Autodesk Fusion 360 part; units mm, degrees
(part 3 of 6)
  line L2235 (12.9289, -30) -> (10, -32.9289)
  line L2236 (13.3431, -31) -> (11, -33.3431)
  line L2237 (16.6569, -31) -> (13.3431, -31)
  line L2238 (19, -33.3431) -> (16.6569, -31)
  line L2239 (19, -36.6569) -> (19, -33.3431)
  line L2240 (16.6569, -39) -> (19, -36.6569)
  line L2241 (13.3431, -39) -> (16.6569, -39)
  line L2242 (11, -36.6569) -> (13.3431, -39)
  line L2243 (11, -33.3431) -> (11, -36.6569)
  line L2244 (10, -37.0711) -> (12.9289, -40)
  line L2245 (12.9289, -40) -> (17.0711, -40)
  line L2246 (17.0711, -40) -> (20, -37.0711)
  line L2247 (20, -37.0711) -> (20, -32.9289)
  line L2248 (20, -32.9289) -> (17.0711, -30)
  line L2249 (20, -32.9289) -> (20, -37.0711)
  line L2250 (22.9289, -30) -> (20, -32.9289)
  line L2251 (23.3431, -31) -> (21, -33.3431)
  line L2252 (26.6569, -31) -> (23.3431, -31)
  line L2253 (29, -33.3431) -> (26.6569, -31)
  line L2254 (29, -36.6569) -> (29, -33.3431)
  line L2255 (26.6569, -39) -> (29, -36.6569)
  line L2256 (23.3431, -39) -> (26.6569, -39)
  line L2257 (21, -36.6569) -> (23.3431, -39)
  line L2258 (21, -33.3431) -> (21, -36.6569)
  line L2259 (20, -37.0711) -> (22.9289, -40)
  line L2260 (22.9289, -40) -> (27.0711, -40)
  line L2261 (27.0711, -40) -> (30, -37.0711)
  line L2262 (30, -37.0711) -> (30, -32.9289)
  line L2263 (30, -32.9289) -> (27.0711, -30)
  line L2264 (30, -32.9289) -> (30, -37.0711)
  line L2265 (32.9289, -30) -> (30, -32.9289)
  line L2266 (33.3431, -31) -> (31, -33.3431)
  line L2267 (36.6569, -31) -> (33.3431, -31)
  line L2268 (39, -33.3431) -> (36.6569, -31)
  line L2269 (39, -36.6569) -> (39, -33.3431)
  line L2270 (36.6569, -39) -> (39, -36.6569)
  line L2271 (33.3431, -39) -> (36.6569, -39)
  line L2272 (31, -36.6569) -> (33.3431, -39)
  line L2273 (31, -33.3431) -> (31, -36.6569)
  line L2274 (30, -37.0711) -> (32.9289, -40)
  line L2275 (32.9289, -40) -> (37.0711, -40)
  line L2276 (37.0711, -40) -> (40, -37.0711)
  line L2277 (40, -37.0711) -> (40, -32.9289)
  line L2278 (40, -32.9289) -> (37.0711, -30)
  line L2279 (40, -32.9289) -> (40, -37.0711)
  line L2280 (42.9289, -30) -> (40, -32.9289)
  line L2281 (43.3431, -31) -> (41, -33.3431)
  line L2282 (46.6569, -31) -> (43.3431, -31)
  line L2283 (49, -33.3431) -> (46.6569, -31)
  line L2284 (49, -36.6569) -> (49, -33.3431)
  line L2285 (46.6569, -39) -> (49, -36.6569)
  line L2286 (43.3431, -39) -> (46.6569, -39)
  line L2287 (41, -36.6569) -> (43.3431, -39)
  line L2288 (41, -33.3431) -> (41, -36.6569)
  line L2289 (40, -37.0711) -> (42.9289, -40)
  line L2290 (42.9289, -40) -> (47.0711, -40)
  line L2291 (47.0711, -40) -> (50, -37.0711)
  line L2292 (50, -37.0711) -> (50, -32.9289)
  line L2293 (50, -32.9289) -> (47.0711, -30)
  line L2294 (50, -32.9289) -> (50, -37.0711)
  line L2295 (52.9289, -30) -> (50, -32.9289)
  line L2296 (53.3431, -31) -> (51, -33.3431)
  line L2297 (56.6569, -31) -> (53.3431, -31)
  line L2298 (59, -33.3431) -> (56.6569, -31)
  line L2299 (59, -36.6569) -> (59, -33.3431)
  line L2300 (56.6569, -39) -> (59, -36.6569)
  line L2301 (53.3431, -39) -> (56.6569, -39)
  line L2302 (51, -36.6569) -> (53.3431, -39)
  line L2303 (51, -33.3431) -> (51, -36.6569)
  line L2304 (50, -37.0711) -> (52.9289, -40)
  line L2305 (52.9289, -40) -> (57.0711, -40)
  line L2306 (57.0711, -40) -> (60, -37.0711)
  line L2307 (60, -37.0711) -> (60, -32.9289)
  line L2308 (60, -32.9289) -> (57.0711, -30)
  line L2309 (60, -32.9289) -> (60, -37.0711)
  line L2310 (62.9289, -30) -> (60, -32.9289)
  line L2311 (63.3431, -31) -> (61, -33.3431)
  line L2312 (66.6569, -31) -> (63.3431, -31)
  line L2313 (69, -33.3431) -> (66.6569, -31)
  line L2314 (69, -36.6569) -> (69, -33.3431)
  line L2315 (66.6569, -39) -> (69, -36.6569)
  line L2316 (63.3431, -39) -> (66.6569, -39)
  line L2317 (61, -36.6569) -> (63.3431, -39)
  line L2318 (61, -33.3431) -> (61, -36.6569)
  line L2319 (60, -37.0711) -> (62.9289, -40)
  line L2320 (62.9289, -40) -> (67.0711, -40)
  line L2321 (67.0711, -40) -> (70, -37.0711)
  line L2322 (70, -37.0711) -> (70, -32.9289)
  line L2323 (70, -32.9289) -> (67.0711, -30)
  line L2324 (-70, -42.9289) -> (-70, -47.0711)
  line L2325 (-67.0711, -40) -> (-70, -42.9289)
  line L2326 (-66.6569, -41) -> (-69, -43.3431)
  line L2327 (-63.3431, -41) -> (-66.6569, -41)
  line L2328 (-61, -43.3431) -> (-63.3431, -41)
  line L2329 (-61, -46.6569) -> (-61, -43.3431)
  line L2330 (-63.3431, -49) -> (-61, -46.6569)
  line L2331 (-66.6569, -49) -> (-63.3431, -49)
  line L2332 (-69, -46.6569) -> (-66.6569, -49)
  line L2333 (-69, -43.3431) -> (-69, -46.6569)
  line L2334 (-70, -47.0711) -> (-67.0711, -50)
  line L2335 (-67.0711, -50) -> (-62.9289, -50)
  line L2336 (-62.9289, -50) -> (-60, -47.0711)
  line L2337 (-60, -47.0711) -> (-60, -42.9289)
  line L2338 (-60, -42.9289) -> (-62.9289, -40)
  line L2339 (-60, -42.9289) -> (-60, -47.0711)
  line L2340 (-57.0711, -40) -> (-60, -42.9289)
  line L2341 (-56.6569, -41) -> (-59, -43.3431)
  line L2342 (-53.3431, -41) -> (-56.6569, -41)
  line L2343 (-51, -43.3431) -> (-53.3431, -41)
  line L2344 (-51, -46.6569) -> (-51, -43.3431)
  line L2345 (-53.3431, -49) -> (-51, -46.6569)
  line L2346 (-56.6569, -49) -> (-53.3431, -49)
  line L2347 (-59, -46.6569) -> (-56.6569, -49)
  line L2348 (-59, -43.3431) -> (-59, -46.6569)
  line L2349 (-60, -47.0711) -> (-57.0711, -50)
  line L2350 (-57.0711, -50) -> (-52.9289, -50)
  line L2351 (-52.9289, -50) -> (-50, -47.0711)
  line L2352 (-50, -47.0711) -> (-50, -42.9289)
  line L2353 (-50, -42.9289) -> (-52.9289, -40)
  line L2354 (-50, -42.9289) -> (-50, -47.0711)
  line L2355 (-47.0711, -40) -> (-50, -42.9289)
  line L2356 (-46.6569, -41) -> (-49, -43.3431)
  line L2357 (-43.3431, -41) -> (-46.6569, -41)
  line L2358 (-41, -43.3431) -> (-43.3431, -41)
  line L2359 (-41, -46.6569) -> (-41, -43.3431)
  line L2360 (-43.3431, -49) -> (-41, -46.6569)
  line L2361 (-46.6569, -49) -> (-43.3431, -49)
  line L2362 (-49, -46.6569) -> (-46.6569, -49)
  line L2363 (-49, -43.3431) -> (-49, -46.6569)
  line L2364 (-50, -47.0711) -> (-47.0711, -50)
  line L2365 (-47.0711, -50) -> (-42.9289, -50)
  line L2366 (-42.9289, -50) -> (-40, -47.0711)
  line L2367 (-40, -47.0711) -> (-40, -42.9289)
  line L2368 (-40, -42.9289) -> (-42.9289, -40)
  line L2369 (-40, -42.9289) -> (-40, -47.0711)
  line L2370 (-37.0711, -40) -> (-40, -42.9289)
  line L2371 (-36.6569, -41) -> (-39, -43.3431)
  line L2372 (-33.3431, -41) -> (-36.6569, -41)
  line L2373 (-31, -43.3431) -> (-33.3431, -41)
  line L2374 (-31, -46.6569) -> (-31, -43.3431)
  line L2375 (-33.3431, -49) -> (-31, -46.6569)
  line L2376 (-36.6569, -49) -> (-33.3431, -49)
  line L2377 (-39, -46.6569) -> (-36.6569, -49)
  line L2378 (-39, -43.3431) -> (-39, -46.6569)
  line L2379 (-40, -47.0711) -> (-37.0711, -50)
  line L2380 (-37.0711, -50) -> (-32.9289, -50)
  line L2381 (-32.9289, -50) -> (-30, -47.0711)
  line L2382 (-30, -47.0711) -> (-30, -42.9289)
  line L2383 (-30, -42.9289) -> (-32.9289, -40)
  line L2384 (-30, -42.9289) -> (-30, -47.0711)
  line L2385 (-27.0711, -40) -> (-30, -42.9289)
  line L2386 (-26.6569, -41) -> (-29, -43.3431)
  line L2387 (-23.3431, -41) -> (-26.6569, -41)
  line L2388 (-21, -43.3431) -> (-23.3431, -41)
  line L2389 (-21, -46.6569) -> (-21, -43.3431)
  line L2390 (-23.3431, -49) -> (-21, -46.6569)
  line L2391 (-26.6569, -49) -> (-23.3431, -49)
  line L2392 (-29, -46.6569) -> (-26.6569, -49)
  line L2393 (-29, -43.3431) -> (-29, -46.6569)
  line L2394 (-30, -47.0711) -> (-27.0711, -50)
  line L2395 (-27.0711, -50) -> (-22.9289, -50)
  line L2396 (-22.9289, -50) -> (-20, -47.0711)
  line L2397 (-20, -47.0711) -> (-20, -42.9289)
  line L2398 (-20, -42.9289) -> (-22.9289, -40)
  line L2399 (-20, -42.9289) -> (-20, -47.0711)
  line L2400 (-17.0711, -40) -> (-20, -42.9289)
  line L2401 (-16.6569, -41) -> (-19, -43.3431)
  line L2402 (-13.3431, -41) -> (-16.6569, -41)
  line L2403 (-11, -43.3431) -> (-13.3431, -41)
  line L2404 (-11, -46.6569) -> (-11, -43.3431)
  line L2405 (-13.3431, -49) -> (-11, -46.6569)
  line L2406 (-16.6569, -49) -> (-13.3431, -49)
  line L2407 (-19, -46.6569) -> (-16.6569, -49)
  line L2408 (-19, -43.3431) -> (-19, -46.6569)
  line L2409 (-20, -47.0711) -> (-17.0711, -50)
  line L2410 (-17.0711, -50) -> (-12.9289, -50)
  line L2411 (-12.9289, -50) -> (-10, -47.0711)
  line L2412 (-10, -47.0711) -> (-10, -42.9289)
  line L2413 (-10, -42.9289) -> (-12.9289, -40)
  line L2414 (-10, -42.9289) -> (-10, -47.0711)
  line L2415 (-7.0711, -40) -> (-10, -42.9289)
  line L2416 (-6.6569, -41) -> (-9, -43.3431)
  line L2417 (-3.3431, -41) -> (-6.6569, -41)
  line L2418 (-1, -43.3431) -> (-3.3431, -41)
  line L2419 (-1, -46.6569) -> (-1, -43.3431)
  line L2420 (-3.3431, -49) -> (-1, -46.6569)
  line L2421 (-6.6569, -49) -> (-3.3431, -49)
  line L2422 (-9, -46.6569) -> (-6.6569, -49)
  line L2423 (-9, -43.3431) -> (-9, -46.6569)
  line L2424 (-10, -47.0711) -> (-7.0711, -50)
  line L2425 (-7.0711, -50) -> (-2.9289, -50)
  line L2426 (-2.9289, -50) -> (0, -47.0711)
  line L2427 (0, -47.0711) -> (0, -42.9289)
  line L2428 (0, -42.9289) -> (-2.9289, -40)
  line L2429 (0, -42.9289) -> (0, -47.0711)
  line L2430 (2.9289, -40) -> (0, -42.9289)
  line L2431 (3.3431, -41) -> (1, -43.3431)
  line L2432 (6.6569, -41) -> (3.3431, -41)
  line L2433 (9, -43.3431) -> (6.6569, -41)
  line L2434 (9, -46.6569) -> (9, -43.3431)
  line L2435 (6.6569, -49) -> (9, -46.6569)
  line L2436 (3.3431, -49) -> (6.6569, -49)
  line L2437 (1, -46.6569) -> (3.3431, -49)
  line L2438 (1, -43.3431) -> (1, -46.6569)
  line L2439 (0, -47.0711) -> (2.9289, -50)
  line L2440 (2.9289, -50) -> (7.0711, -50)
  line L2441 (7.0711, -50) -> (10, -47.0711)
  line L2442 (10, -47.0711) -> (10, -42.9289)
  line L2443 (10, -42.9289) -> (7.0711, -40)
  line L2444 (10, -42.9289) -> (10, -47.0711)
  line L2445 (12.9289, -40) -> (10, -42.9289)
  line L2446 (13.3431, -41) -> (11, -43.3431)
  line L2447 (16.6569, -41) -> (13.3431, -41)
  line L2448 (19, -43.3431) -> (16.6569, -41)
  line L2449 (19, -46.6569) -> (19, -43.3431)
  line L2450 (16.6569, -49) -> (19, -46.6569)
  line L2451 (13.3431, -49) -> (16.6569, -49)
  line L2452 (11, -46.6569) -> (13.3431, -49)
  line L2453 (11, -43.3431) -> (11, -46.6569)
  line L2454 (10, -47.0711) -> (12.9289, -50)
  line L2455 (12.9289, -50) -> (17.0711, -50)
  line L2456 (17.0711, -50) -> (20, -47.0711)
  line L2457 (20, -47.0711) -> (20, -42.9289)
  line L2458 (20, -42.9289) -> (17.0711, -40)
  line L2459 (20, -42.9289) -> (20, -47.0711)
  line L2460 (22.9289, -40) -> (20, -42.9289)
  line L2461 (23.3431, -41) -> (21, -43.3431)
  line L2462 (26.6569, -41) -> (23.3431, -41)
  line L2463 (29, -43.3431) -> (26.6569, -41)
  line L2464 (29, -46.6569) -> (29, -43.3431)
  line L2465 (26.6569, -49) -> (29, -46.6569)
  line L2466 (23.3431, -49) -> (26.6569, -49)
  line L2467 (21, -46.6569) -> (23.3431, -49)
  line L2468 (21, -43.3431) -> (21, -46.6569)
  line L2469 (20, -47.0711) -> (22.9289, -50)
  line L2470 (22.9289, -50) -> (27.0711, -50)
  line L2471 (27.0711, -50) -> (30, -47.0711)
  line L2472 (30, -47.0711) -> (30, -42.9289)
  line L2473 (30, -42.9289) -> (27.0711, -40)
  line L2474 (30, -42.9289) -> (30, -47.0711)
  line L2475 (32.9289, -40) -> (30, -42.9289)
  line L2476 (33.3431, -41) -> (31, -43.3431)
  line L2477 (36.6569, -41) -> (33.3431, -41)
  line L2478 (39, -43.3431) -> (36.6569, -41)
  line L2479 (39, -46.6569) -> (39, -43.3431)
  line L2480 (36.6569, -49) -> (39, -46.6569)
  line L2481 (33.3431, -49) -> (36.6569, -49)
  line L2482 (31, -46.6569) -> (33.3431, -49)
  line L2483 (31, -43.3431) -> (31, -46.6569)
  line L2484 (30, -47.0711) -> (32.9289, -50)
  line L2485 (32.9289, -50) -> (37.0711, -50)
  line L2486 (37.0711, -50) -> (40, -47.0711)
  line L2487 (40, -47.0711) -> (40, -42.9289)
  line L2488 (40, -42.9289) -> (37.0711, -40)
  line L2489 (40, -42.9289) -> (40, -47.0711)
  line L2490 (42.9289, -40) -> (40, -42.9289)
  line L2491 (43.3431, -41) -> (41, -43.3431)
  line L2492 (46.6569, -41) -> (43.3431, -41)
  line L2493 (49, -43.3431) -> (46.6569, -41)
  line L2494 (49, -46.6569) -> (49, -43.3431)
  line L2495 (46.6569, -49) -> (49, -46.6569)
  line L2496 (43.3431, -49) -> (46.6569, -49)
  line L2497 (41, -46.6569) -> (43.3431, -49)
  line L2498 (41, -43.3431) -> (41, -46.6569)
  line L2499 (40, -47.0711) -> (42.9289, -50)
  line L2500 (42.9289, -50) -> (47.0711, -50)
  line L2501 (47.0711, -50) -> (50, -47.0711)
  line L2502 (50, -47.0711) -> (50, -42.9289)
  line L2503 (50, -42.9289) -> (47.0711, -40)
  line L2504 (50, -42.9289) -> (50, -47.0711)
  line L2505 (52.9289, -40) -> (50, -42.9289)
  line L2506 (53.3431, -41) -> (51, -43.3431)
  line L2507 (56.6569, -41) -> (53.3431, -41)
  line L2508 (59, -43.3431) -> (56.6569, -41)
  line L2509 (59, -46.6569) -> (59, -43.3431)
  line L2510 (56.6569, -49) -> (59, -46.6569)
  line L2511 (53.3431, -49) -> (56.6569, -49)
  line L2512 (51, -46.6569) -> (53.3431, -49)
  line L2513 (51, -43.3431) -> (51, -46.6569)
  line L2514 (50, -47.0711) -> (52.9289, -50)
  line L2515 (52.9289, -50) -> (57.0711, -50)
  line L2516 (57.0711, -50) -> (60, -47.0711)
  line L2517 (60, -47.0711) -> (60, -42.9289)
  line L2518 (60, -42.9289) -> (57.0711, -40)
  line L2519 (60, -42.9289) -> (60, -47.0711)
  line L2520 (62.9289, -40) -> (60, -42.9289)
  line L2521 (63.3431, -41) -> (61, -43.3431)
  line L2522 (66.6569, -41) -> (63.3431, -41)
  line L2523 (69, -43.3431) -> (66.6569, -41)
  line L2524 (69, -46.6569) -> (69, -43.3431)
  line L2525 (66.6569, -49) -> (69, -46.6569)
  line L2526 (63.3431, -49) -> (66.6569, -49)
  line L2527 (61, -46.6569) -> (63.3431, -49)
  line L2528 (61, -43.3431) -> (61, -46.6569)
  line L2529 (60, -47.0711) -> (62.9289, -50)
  line L2530 (62.9289, -50) -> (67.0711, -50)
  line L2531 (67.0711, -50) -> (70, -47.0711)
  line L2532 (70, -47.0711) -> (70, -42.9289)
  line L2533 (70, -42.9289) -> (67.0711, -40)
  line L2534 (-70, -52.9289) -> (-70, -57.0711)
  line L2535 (-67.0711, -50) -> (-70, -52.9289)
  line L2536 (-66.6569, -51) -> (-69, -53.3431)
  line L2537 (-63.3431, -51) -> (-66.6569, -51)
  line L2538 (-61, -53.3431) -> (-63.3431, -51)
  line L2539 (-61, -56.6569) -> (-61, -53.3431)
  line L2540 (-63.3431, -59) -> (-61, -56.6569)
  line L2541 (-66.6569, -59) -> (-63.3431, -59)
  line L2542 (-69, -56.6569) -> (-66.6569, -59)
  line L2543 (-69, -53.3431) -> (-69, -56.6569)
  line L2544 (-70, -57.0711) -> (-67.0711, -60)
  line L2545 (-67.0711, -60) -> (-62.9289, -60)
  line L2546 (-62.9289, -60) -> (-60, -57.0711)
  line L2547 (-60, -57.0711) -> (-60, -52.9289)
  line L2548 (-60, -52.9289) -> (-62.9289, -50)
  line L2549 (-60, -52.9289) -> (-60, -57.0711)
  line L2550 (-57.0711, -50) -> (-60, -52.9289)
  line L2551 (-56.6569, -51) -> (-59, -53.3431)
  line L2552 (-53.3431, -51) -> (-56.6569, -51)
  line L2553 (-51, -53.3431) -> (-53.3431, -51)
  line L2554 (-51, -56.6569) -> (-51, -53.3431)
  line L2555 (-53.3431, -59) -> (-51, -56.6569)
  line L2556 (-56.6569, -59) -> (-53.3431, -59)
  line L2557 (-59, -56.6569) -> (-56.6569, -59)
  line L2558 (-59, -53.3431) -> (-59, -56.6569)
  line L2559 (-60, -57.0711) -> (-57.0711, -60)
  line L2560 (-57.0711, -60) -> (-52.9289, -60)
  line L2561 (-52.9289, -60) -> (-50, -57.0711)
  line L2562 (-50, -57.0711) -> (-50, -52.9289)
  line L2563 (-50, -52.9289) -> (-52.9289, -50)
  line L2564 (-50, -52.9289) -> (-50, -57.0711)
  line L2565 (-47.0711, -50) -> (-50, -52.9289)
  line L2566 (-46.6569, -51) -> (-49, -53.3431)
  line L2567 (-43.3431, -51) -> (-46.6569, -51)
  line L2568 (-41, -53.3431) -> (-43.3431, -51)
  line L2569 (-41, -56.6569) -> (-41, -53.3431)
  line L2570 (-43.3431, -59) -> (-41, -56.6569)
  line L2571 (-46.6569, -59) -> (-43.3431, -59)
  line L2572 (-49, -56.6569) -> (-46.6569, -59)
  line L2573 (-49, -53.3431) -> (-49, -56.6569)
  line L2574 (-50, -57.0711) -> (-47.0711, -60)
  line L2575 (-47.0711, -60) -> (-42.9289, -60)
  line L2576 (-42.9289, -60) -> (-40, -57.0711)
  line L2577 (-40, -57.0711) -> (-40, -52.9289)
  line L2578 (-40, -52.9289) -> (-42.9289, -50)
  line L2579 (-40, -52.9289) -> (-40, -57.0711)
  line L2580 (-37.0711, -50) -> (-40, -52.9289)
  line L2581 (-36.6569, -51) -> (-39, -53.3431)
  line L2582 (-33.3431, -51) -> (-36.6569, -51)
  line L2583 (-31, -53.3431) -> (-33.3431, -51)
  line L2584 (-31, -56.6569) -> (-31, -53.3431)
  line L2585 (-33.3431, -59) -> (-31, -56.6569)
  line L2586 (-36.6569, -59) -> (-33.3431, -59)
  line L2587 (-39, -56.6569) -> (-36.6569, -59)
  line L2588 (-39, -53.3431) -> (-39, -56.6569)
  line L2589 (-40, -57.0711) -> (-37.0711, -60)
  line L2590 (-37.0711, -60) -> (-32.9289, -60)
  line L2591 (-32.9289, -60) -> (-30, -57.0711)
  line L2592 (-30, -57.0711) -> (-30, -52.9289)
  line L2593 (-30, -52.9289) -> (-32.9289, -50)
  line L2594 (-30, -52.9289) -> (-30, -57.0711)
  line L2595 (-27.0711, -50) -> (-30, -52.9289)
  line L2596 (-26.6569, -51) -> (-29, -53.3431)
  line L2597 (-23.3431, -51) -> (-26.6569, -51)
  line L2598 (-21, -53.3431) -> (-23.3431, -51)
  line L2599 (-21, -56.6569) -> (-21, -53.3431)
  line L2600 (-23.3431, -59) -> (-21, -56.6569)
  line L2601 (-26.6569, -59) -> (-23.3431, -59)
  line L2602 (-29, -56.6569) -> (-26.6569, -59)
  line L2603 (-29, -53.3431) -> (-29, -56.6569)
  line L2604 (-30, -57.0711) -> (-27.0711, -60)
  line L2605 (-27.0711, -60) -> (-22.9289, -60)
  line L2606 (-22.9289, -60) -> (-20, -57.0711)
  line L2607 (-20, -57.0711) -> (-20, -52.9289)
  line L2608 (-20, -52.9289) -> (-22.9289, -50)
  line L2609 (-20, -52.9289) -> (-20, -57.0711)
  line L2610 (-17.0711, -50) -> (-20, -52.9289)
  line L2611 (-16.6569, -51) -> (-19, -53.3431)
  line L2612 (-13.3431, -51) -> (-16.6569, -51)
  line L2613 (-11, -53.3431) -> (-13.3431, -51)
  line L2614 (-11, -56.6569) -> (-11, -53.3431)
  line L2615 (-13.3431, -59) -> (-11, -56.6569)
  line L2616 (-16.6569, -59) -> (-13.3431, -59)
  line L2617 (-19, -56.6569) -> (-16.6569, -59)
  line L2618 (-19, -53.3431) -> (-19, -56.6569)
  line L2619 (-20, -57.0711) -> (-17.0711, -60)
  line L2620 (-17.0711, -60) -> (-12.9289, -60)
  line L2621 (-12.9289, -60) -> (-10, -57.0711)
  line L2622 (-10, -57.0711) -> (-10, -52.9289)
  line L2623 (-10, -52.9289) -> (-12.9289, -50)
  line L2624 (-10, -52.9289) -> (-10, -57.0711)
  line L2625 (-7.0711, -50) -> (-10, -52.9289)
  line L2626 (-6.6569, -51) -> (-9, -53.3431)
  line L2627 (-3.3431, -51) -> (-6.6569, -51)
  line L2628 (-1, -53.3431) -> (-3.3431, -51)
  line L2629 (-1, -56.6569) -> (-1, -53.3431)
  line L2630 (-3.3431, -59) -> (-1, -56.6569)
  line L2631 (-6.6569, -59) -> (-3.3431, -59)
  line L2632 (-9, -56.6569) -> (-6.6569, -59)
  line L2633 (-9, -53.3431) -> (-9, -56.6569)
  line L2634 (-10, -57.0711) -> (-7.0711, -60)
  line L2635 (-7.0711, -60) -> (-2.9289, -60)
  line L2636 (-2.9289, -60) -> (0, -57.0711)
  line L2637 (0, -57.0711) -> (0, -52.9289)
  line L2638 (0, -52.9289) -> (-2.9289, -50)
  line L2639 (0, -52.9289) -> (0, -57.0711)
  line L2640 (2.9289, -50) -> (0, -52.9289)
  line L2641 (3.3431, -51) -> (1, -53.3431)
  line L2642 (6.6569, -51) -> (3.3431, -51)
  line L2643 (9, -53.3431) -> (6.6569, -51)
  line L2644 (9, -56.6569) -> (9, -53.3431)
  line L2645 (6.6569, -59) -> (9, -56.6569)
  line L2646 (3.3431, -59) -> (6.6569, -59)
  line L2647 (1, -56.6569) -> (3.3431, -59)
  line L2648 (1, -53.3431) -> (1, -56.6569)
  line L2649 (0, -57.0711) -> (2.9289, -60)
  line L2650 (2.9289, -60) -> (7.0711, -60)
  line L2651 (7.0711, -60) -> (10, -57.0711)
  line L2652 (10, -57.0711) -> (10, -52.9289)
  line L2653 (10, -52.9289) -> (7.0711, -50)
  line L2654 (10, -52.9289) -> (10, -57.0711)
  line L2655 (12.9289, -50) -> (10, -52.9289)
  line L2656 (13.3431, -51) -> (11, -53.3431)
  line L2657 (16.6569, -51) -> (13.3431, -51)
  line L2658 (19, -53.3431) -> (16.6569, -51)
  line L2659 (19, -56.6569) -> (19, -53.3431)
  line L2660 (16.6569, -59) -> (19, -56.6569)
  line L2661 (13.3431, -59) -> (16.6569, -59)
  line L2662 (11, -56.6569) -> (13.3431, -59)
  line L2663 (11, -53.3431) -> (11, -56.6569)
  line L2664 (10, -57.0711) -> (12.9289, -60)
  line L2665 (12.9289, -60) -> (17.0711, -60)
  line L2666 (17.0711, -60) -> (20, -57.0711)
  line L2667 (20, -57.0711) -> (20, -52.9289)
  line L2668 (20, -52.9289) -> (17.0711, -50)
  line L2669 (20, -52.9289) -> (20, -57.0711)
  line L2670 (22.9289, -50) -> (20, -52.9289)
  line L2671 (23.3431, -51) -> (21, -53.3431)
  line L2672 (26.6569, -51) -> (23.3431, -51)
  line L2673 (29, -53.3431) -> (26.6569, -51)
  line L2674 (29, -56.6569) -> (29, -53.3431)
  line L2675 (26.6569, -59) -> (29, -56.6569)
  line L2676 (23.3431, -59) -> (26.6569, -59)
  line L2677 (21, -56.6569) -> (23.3431, -59)
  line L2678 (21, -53.3431) -> (21, -56.6569)
  line L2679 (20, -57.0711) -> (22.9289, -60)
  line L2680 (22.9289, -60) -> (27.0711, -60)
  line L2681 (27.0711, -60) -> (30, -57.0711)
  line L2682 (30, -57.0711) -> (30, -52.9289)
  line L2683 (30, -52.9289) -> (27.0711, -50)
  line L2684 (30, -52.9289) -> (30, -57.0711)
  line L2685 (32.9289, -50) -> (30, -52.9289)
  line L2686 (33.3431, -51) -> (31, -53.3431)
  line L2687 (36.6569, -51) -> (33.3431, -51)
  line L2688 (39, -53.3431) -> (36.6569, -51)
  line L2689 (39, -56.6569) -> (39, -53.3431)
  line L2690 (36.6569, -59) -> (39, -56.6569)
  line L2691 (33.3431, -59) -> (36.6569, -59)
  line L2692 (31, -56.6569) -> (33.3431, -59)
  line L2693 (31, -53.3431) -> (31, -56.6569)
  line L2694 (30, -57.0711) -> (32.9289, -60)
  line L2695 (32.9289, -60) -> (37.0711, -60)
  line L2696 (37.0711, -60) -> (40, -57.0711)
  line L2697 (40, -57.0711) -> (40, -52.9289)
  line L2698 (40, -52.9289) -> (37.0711, -50)
  line L2699 (40, -52.9289) -> (40, -57.0711)
  line L2700 (42.9289, -50) -> (40, -52.9289)
  line L2701 (43.3431, -51) -> (41, -53.3431)
  line L2702 (46.6569, -51) -> (43.3431, -51)
  line L2703 (49, -53.3431) -> (46.6569, -51)
  line L2704 (49, -56.6569) -> (49, -53.3431)
  line L2705 (46.6569, -59) -> (49, -56.6569)
  line L2706 (43.3431, -59) -> (46.6569, -59)
  line L2707 (41, -56.6569) -> (43.3431, -59)
  line L2708 (41, -53.3431) -> (41, -56.6569)
  line L2709 (40, -57.0711) -> (42.9289, -60)
  line L2710 (42.9289, -60) -> (47.0711, -60)
  line L2711 (47.0711, -60) -> (50, -57.0711)
  line L2712 (50, -57.0711) -> (50, -52.9289)
  line L2713 (50, -52.9289) -> (47.0711, -50)
  line L2714 (50, -52.9289) -> (50, -57.0711)
  line L2715 (52.9289, -50) -> (50, -52.9289)
  line L2716 (53.3431, -51) -> (51, -53.3431)
  line L2717 (56.6569, -51) -> (53.3431, -51)
  line L2718 (59, -53.3431) -> (56.6569, -51)
  line L2719 (59, -56.6569) -> (59, -53.3431)
  line L2720 (56.6569, -59) -> (59, -56.6569)
  line L2721 (53.3431, -59) -> (56.6569, -59)
  line L2722 (51, -56.6569) -> (53.3431, -59)
  line L2723 (51, -53.3431) -> (51, -56.6569)
  line L2724 (50, -57.0711) -> (52.9289, -60)
  line L2725 (52.9289, -60) -> (57.0711, -60)
  line L2726 (57.0711, -60) -> (60, -57.0711)
  line L2727 (60, -57.0711) -> (60, -52.9289)
  line L2728 (60, -52.9289) -> (57.0711, -50)
  line L2729 (60, -52.9289) -> (60, -57.0711)
  line L2730 (62.9289, -50) -> (60, -52.9289)
  line L2731 (63.3431, -51) -> (61, -53.3431)
  line L2732 (66.6569, -51) -> (63.3431, -51)
  line L2733 (69, -53.3431) -> (66.6569, -51)
  line L2734 (69, -56.6569) -> (69, -53.3431)
  line L2735 (66.6569, -59) -> (69, -56.6569)
  line L2736 (63.3431, -59) -> (66.6569, -59)
  line L2737 (61, -56.6569) -> (63.3431, -59)
  line L2738 (61, -53.3431) -> (61, -56.6569)
  line L2739 (60, -57.0711) -> (62.9289, -60)
  line L2740 (62.9289, -60) -> (67.0711, -60)
  line L2741 (67.0711, -60) -> (70, -57.0711)
  line L2742 (70, -57.0711) -> (70, -52.9289)
  line L2743 (70, -52.9289) -> (67.0711, -50)
  line L2744 (-70, -62.9289) -> (-70, -67.0711)
  line L2745 (-67.0711, -60) -> (-70, -62.9289)
  line L2746 (-66.6569, -61) -> (-69, -63.3431)
  line L2747 (-63.3431, -61) -> (-66.6569, -61)
  line L2748 (-61, -63.3431) -> (-63.3431, -61)
  line L2749 (-61, -66.6569) -> (-61, -63.3431)
  line L2750 (-63.3431, -69) -> (-61, -66.6569)
  line L2751 (-66.6569, -69) -> (-63.3431, -69)
  line L2752 (-69, -66.6569) -> (-66.6569, -69)
  line L2753 (-69, -63.3431) -> (-69, -66.6569)
  line L2754 (-70, -67.0711) -> (-67.0711, -70)
  line L2755 (-67.0711, -70) -> (-62.9289, -70)
  line L2756 (-62.9289, -70) -> (-60, -67.0711)
  line L2757 (-60, -67.0711) -> (-60, -62.9289)
  line L2758 (-60, -62.9289) -> (-62.9289, -60)
  line L2759 (-60, -62.9289) -> (-60, -67.0711)
  line L2760 (-57.0711, -60) -> (-60, -62.9289)
  line L2761 (-56.6569, -61) -> (-59, -63.3431)
  line L2762 (-53.3431, -61) -> (-56.6569, -61)
  line L2763 (-51, -63.3431) -> (-53.3431, -61)
  line L2764 (-51, -66.6569) -> (-51, -63.3431)
  line L2765 (-53.3431, -69) -> (-51, -66.6569)
  line L2766 (-56.6569, -69) -> (-53.3431, -69)
  line L2767 (-59, -66.6569) -> (-56.6569, -69)
  line L2768 (-59, -63.3431) -> (-59, -66.6569)
  line L2769 (-60, -67.0711) -> (-57.0711, -70)
  line L2770 (-57.0711, -70) -> (-52.9289, -70)
  line L2771 (-52.9289, -70) -> (-50, -67.0711)
  line L2772 (-50, -67.0711) -> (-50, -62.9289)
  line L2773 (-50, -62.9289) -> (-52.9289, -60)
  line L2774 (-50, -62.9289) -> (-50, -67.0711)
  line L2775 (-47.0711, -60) -> (-50, -62.9289)
  line L2776 (-46.6569, -61) -> (-49, -63.3431)
  line L2777 (-43.3431, -61) -> (-46.6569, -61)
  line L2778 (-41, -63.3431) -> (-43.3431, -61)
  line L2779 (-41, -66.6569) -> (-41, -63.3431)
  line L2780 (-43.3431, -69) -> (-41, -66.6569)
  line L2781 (-46.6569, -69) -> (-43.3431, -69)
  line L2782 (-49, -66.6569) -> (-46.6569, -69)
  line L2783 (-49, -63.3431) -> (-49, -66.6569)
  line L2784 (-50, -67.0711) -> (-47.0711, -70)
  line L2785 (-47.0711, -70) -> (-42.9289, -70)
  line L2786 (-42.9289, -70) -> (-40, -67.0711)
  line L2787 (-40, -67.0711) -> (-40, -62.9289)
  line L2788 (-40, -62.9289) -> (-42.9289, -60)
  line L2789 (-40, -62.9289) -> (-40, -67.0711)
  line L2790 (-37.0711, -60) -> (-40, -62.9289)
  line L2791 (-36.6569, -61) -> (-39, -63.3431)
  line L2792 (-33.3431, -61) -> (-36.6569, -61)
  line L2793 (-31, -63.3431) -> (-33.3431, -61)
  line L2794 (-31, -66.6569) -> (-31, -63.3431)
  line L2795 (-33.3431, -69) -> (-31, -66.6569)
  line L2796 (-36.6569, -69) -> (-33.3431, -69)
  line L2797 (-39, -66.6569) -> (-36.6569, -69)
  line L2798 (-39, -63.3431) -> (-39, -66.6569)
  line L2799 (-40, -67.0711) -> (-37.0711, -70)
  line L2800 (-37.0711, -70) -> (-32.9289, -70)
  line L2801 (-32.9289, -70) -> (-30, -67.0711)
  line L2802 (-30, -67.0711) -> (-30, -62.9289)
  line L2803 (-30, -62.9289) -> (-32.9289, -60)
  line L2804 (-30, -62.9289) -> (-30, -67.0711)
  line L2805 (-27.0711, -60) -> (-30, -62.9289)
  line L2806 (-26.6569, -61) -> (-29, -63.3431)
  line L2807 (-23.3431, -61) -> (-26.6569, -61)
  line L2808 (-21, -63.3431) -> (-23.3431, -61)
  line L2809 (-21, -66.6569) -> (-21, -63.3431)
  line L2810 (-23.3431, -69) -> (-21, -66.6569)
  line L2811 (-26.6569, -69) -> (-23.3431, -69)
  line L2812 (-29, -66.6569) -> (-26.6569, -69)
  line L2813 (-29, -63.3431) -> (-29, -66.6569)
  line L2814 (-30, -67.0711) -> (-27.0711, -70)
  line L2815 (-27.0711, -70) -> (-22.9289, -70)
  line L2816 (-22.9289, -70) -> (-20, -67.0711)
  line L2817 (-20, -67.0711) -> (-20, -62.9289)
  line L2818 (-20, -62.9289) -> (-22.9289, -60)
  line L2819 (-20, -62.9289) -> (-20, -67.0711)
  line L2820 (-17.0711, -60) -> (-20, -62.9289)
  line L2821 (-16.6569, -61) -> (-19, -63.3431)
  line L2822 (-13.3431, -61) -> (-16.6569, -61)
  line L2823 (-11, -63.3431) -> (-13.3431, -61)
  line L2824 (-11, -66.6569) -> (-11, -63.3431)
  line L2825 (-13.3431, -69) -> (-11, -66.6569)
  line L2826 (-16.6569, -69) -> (-13.3431, -69)
  line L2827 (-19, -66.6569) -> (-16.6569, -69)
  line L2828 (-19, -63.3431) -> (-19, -66.6569)
  line L2829 (-20, -67.0711) -> (-17.0711, -70)
  line L2830 (-17.0711, -70) -> (-12.9289, -70)
  line L2831 (-12.9289, -70) -> (-10, -67.0711)
  line L2832 (-10, -67.0711) -> (-10, -62.9289)
  line L2833 (-10, -62.9289) -> (-12.9289, -60)
  line L2834 (-10, -62.9289) -> (-10, -67.0711)
  line L2835 (-7.0711, -60) -> (-10, -62.9289)
  line L2836 (-6.6569, -61) -> (-9, -63.3431)
  line L2837 (-3.3431, -61) -> (-6.6569, -61)
  line L2838 (-1, -63.3431) -> (-3.3431, -61)
  line L2839 (-1, -66.6569) -> (-1, -63.3431)
  line L2840 (-3.3431, -69) -> (-1, -66.6569)
  line L2841 (-6.6569, -69) -> (-3.3431, -69)
  line L2842 (-9, -66.6569) -> (-6.6569, -69)
  line L2843 (-9, -63.3431) -> (-9, -66.6569)
  line L2844 (-10, -67.0711) -> (-7.0711, -70)
  line L2845 (-7.0711, -70) -> (-2.9289, -70)
  line L2846 (-2.9289, -70) -> (0, -67.0711)
  line L2847 (0, -67.0711) -> (0, -62.9289)
  line L2848 (0, -62.9289) -> (-2.9289, -60)
  line L2849 (0, -62.9289) -> (0, -67.0711)
  line L2850 (2.9289, -60) -> (0, -62.9289)
  line L2851 (3.3431, -61) -> (1, -63.3431)
  line L2852 (6.6569, -61) -> (3.3431, -61)
  line L2853 (9, -63.3431) -> (6.6569, -61)
  line L2854 (9, -66.6569) -> (9, -63.3431)
  line L2855 (6.6569, -69) -> (9, -66.6569)
  line L2856 (3.3431, -69) -> (6.6569, -69)
  line L2857 (1, -66.6569) -> (3.3431, -69)
  line L2858 (1, -63.3431) -> (1, -66.6569)
  line L2859 (0, -67.0711) -> (2.9289, -70)
  line L2860 (2.9289, -70) -> (7.0711, -70)
  line L2861 (7.0711, -70) -> (10, -67.0711)
  line L2862 (10, -67.0711) -> (10, -62.9289)
  line L2863 (10, -62.9289) -> (7.0711, -60)
  line L2864 (10, -62.9289) -> (10, -67.0711)
  line L2865 (12.9289, -60) -> (10, -62.9289)
  line L2866 (13.3431, -61) -> (11, -63.3431)
  line L2867 (16.6569, -61) -> (13.3431, -61)
  line L2868 (19, -63.3431) -> (16.6569, -61)
  line L2869 (19, -66.6569) -> (19, -63.3431)
  line L2870 (16.6569, -69) -> (19, -66.6569)
  line L2871 (13.3431, -69) -> (16.6569, -69)
  line L2872 (11, -66.6569) -> (13.3431, -69)
  line L2873 (11, -63.3431) -> (11, -66.6569)
  line L2874 (10, -67.0711) -> (12.9289, -70)
  line L2875 (12.9289, -70) -> (17.0711, -70)
  line L2876 (17.0711, -70) -> (20, -67.0711)
  line L2877 (20, -67.0711) -> (20, -62.9289)
  line L2878 (20, -62.9289) -> (17.0711, -60)
  line L2879 (20, -62.9289) -> (20, -67.0711)
  line L2880 (22.9289, -60) -> (20, -62.9289)
  line L2881 (23.3431, -61) -> (21, -63.3431)
  line L2882 (26.6569, -61) -> (23.3431, -61)
  line L2883 (29, -63.3431) -> (26.6569, -61)
  line L2884 (29, -66.6569) -> (29, -63.3431)
  line L2885 (26.6569, -69) -> (29, -66.6569)
  line L2886 (23.3431, -69) -> (26.6569, -69)
  line L2887 (21, -66.6569) -> (23.3431, -69)
  line L2888 (21, -63.3431) -> (21, -66.6569)
  line L2889 (20, -67.0711) -> (22.9289, -70)
  line L2890 (22.9289, -70) -> (27.0711, -70)
  line L2891 (27.0711, -70) -> (30, -67.0711)
  line L2892 (30, -67.0711) -> (30, -62.9289)
  line L2893 (30, -62.9289) -> (27.0711, -60)
  line L2894 (30, -62.9289) -> (30, -67.0711)
  line L2895 (32.9289, -60) -> (30, -62.9289)
  line L2896 (33.3431, -61) -> (31, -63.3431)
  line L2897 (36.6569, -61) -> (33.3431, -61)
  line L2898 (39, -63.3431) -> (36.6569, -61)
  line L2899 (39, -66.6569) -> (39, -63.3431)
  line L2900 (36.6569, -69) -> (39, -66.6569)
  line L2901 (33.3431, -69) -> (36.6569, -69)
  line L2902 (31, -66.6569) -> (33.3431, -69)
  line L2903 (31, -63.3431) -> (31, -66.6569)
  line L2904 (30, -67.0711) -> (32.9289, -70)
  line L2905 (32.9289, -70) -> (37.0711, -70)
  line L2906 (37.0711, -70) -> (40, -67.0711)
  line L2907 (40, -67.0711) -> (40, -62.9289)
  line L2908 (40, -62.9289) -> (37.0711, -60)
  line L2909 (40, -62.9289) -> (40, -67.0711)
  line L2910 (42.9289, -60) -> (40, -62.9289)
  line L2911 (43.3431, -61) -> (41, -63.3431)
  line L2912 (46.6569, -61) -> (43.3431, -61)
  line L2913 (49, -63.3431) -> (46.6569, -61)
  line L2914 (49, -66.6569) -> (49, -63.3431)
  line L2915 (46.6569, -69) -> (49, -66.6569)
  line L2916 (43.3431, -69) -> (46.6569, -69)
  line L2917 (41, -66.6569) -> (43.3431, -69)
  line L2918 (41, -63.3431) -> (41, -66.6569)
  line L2919 (40, -67.0711) -> (42.9289, -70)
  line L2920 (42.9289, -70) -> (47.0711, -70)
  line L2921 (47.0711, -70) -> (50, -67.0711)
  line L2922 (50, -67.0711) -> (50, -62.9289)
  line L2923 (50, -62.9289) -> (47.0711, -60)
  line L2924 (50, -62.9289) -> (50, -67.0711)
  line L2925 (52.9289, -60) -> (50, -62.9289)
  line L2926 (53.3431, -61) -> (51, -63.3431)
  line L2927 (56.6569, -61) -> (53.3431, -61)
  line L2928 (59, -63.3431) -> (56.6569, -61)
  line L2929 (59, -66.6569) -> (59, -63.3431)
  line L2930 (56.6569, -69) -> (59, -66.6569)
  line L2931 (53.3431, -69) -> (56.6569, -69)
  line L2932 (51, -66.6569) -> (53.3431, -69)
  line L2933 (51, -63.3431) -> (51, -66.6569)
  line L2934 (50, -67.0711) -> (52.9289, -70)
  line L2935 (52.9289, -70) -> (57.0711, -70)
  line L2936 (57.0711, -70) -> (60, -67.0711)
  line L2937 (60, -67.0711) -> (60, -62.9289)
  line L2938 (60, -62.9289) -> (57.0711, -60)
  line L2939 (60, -62.9289) -> (60, -67.0711)
  line L2940 (62.9289, -60) -> (60, -62.9289)
  line L2941 (63.3431, -61) -> (61, -63.3431)
  line L2942 (66.6569, -61) -> (63.3431, -61)
  line L2943 (69, -63.3431) -> (66.6569, -61)
  line L2944 (69, -66.6569) -> (69, -63.3431)
  line L2945 (66.6569, -69) -> (69, -66.6569)
  line L2946 (63.3431, -69) -> (66.6569, -69)
  line L2947 (61, -66.6569) -> (63.3431, -69)
  line L2948 (61, -63.3431) -> (61, -66.6569)
  line L2949 (60, -67.0711) -> (62.9289, -70)
  line L2950 (62.9289, -70) -> (67.0711, -70)
  line L2951 (67.0711, -70) -> (70, -67.0711)
  line L2952 (70, -67.0711) -> (70, -62.9289)
  line L2953 (70, -62.9289) -> (67.0711, -60)
  point P0 (-65, 65)
  point P1 (-65, 65)
  dimension "d1" = 150
  dimension "d2" = 150
  dimension "d3" = 140
  dimension "d4" = 140
  dimension "d5" = 10
  dimension "d6" = 4
  dimension "d11" = 10
  dimension "d12" = -10
  constraint horizontal L0
  constraint perpendicular L0 L1
  constraint parallel L0 L2
  constraint parallel L1 L3
  constraint coincident L4 origin
  constraint coincident L5 origin
  constraint horizontal L6
  constraint perpendicular L6 L7
  constraint parallel L6 L8
  constraint parallel L7 L9
  constraint coincident L10 origin
  constraint coincident L11 origin
  constraint perpendicular L9 L12
  constraint coincident L10 P1
  constraint coincident P1 P0
  measures "d1" distance of L1.end L2.end
  measures "d2" distance of L0.end L1.end
  measures "d3" distance of L7.end L8.end
  measures "d4" distance of L6.end L7.end
  measures "d5" distance of L6.start L12.end
  measures "d6" distance of P1 L28
extrude "Extrude1" add sketch "Sketch1" along normal blind 1 contours L0 L1 L2 L3 | L6 L9 L12 L13 L14 L15 L16 L17 L18 L19 L20 L29
extrude "Extrude2" add sketch "Sketch1" along normal blind 1 contours L6 L14 L29 L30 L39 L40 L41 L42 L43 L44 | L9 L20 L224 L225 L234 L235 L236 L237 L238 L239 | L40 L237 L239 L240 L249 L250 L251 L252 L253 L254 | L9 L235 L434 L435 L444 L445 L446 L447 L448 L449 | L6 L42 L44 L45 L54 L55 L56 L57 L58 L59 | L55 L252 L254 L255 L264 L265 L266 L267 L268 L269 | L9 L445 L644 L645 L654 L655 L656 L657 L658 L659 | L250 L447 L449 L450 L459 L460 L461 L462 L463 L464 | L6 L57 L59 L60 L69 L70 L71 L72 L73 L74 | L265 L462 L464 L465 L474 L475 L476 L477 L478 L479 | L9 L655 L854 L855 L864 L865 L866 L867 L868 L869 | L460 L657 L659 L660 L669 L670 L671 L672 L673 L674 | L6 L72 L74 L75 L84 L85 L86 L87 L88 L89 | L70 L267 L269 L270 L279 L280 L281 L282 L283 L284 | L280 L477 L479 L480 L489 L490 L491 L492 L493 L494 | L9 L865 L1064 L1065 L1074 L1075 L1076 L1077 L1078 L1079 | L670 L867 L869 L870 L879 L880 L881 L882 L883 L884 | L475 L672 L674 L675 L684 L685 L686 L687 L688 L689 | L6 L87 L89 L90 L99 L100 L101 L102 L103 L104 | L85 L282 L284 L285 L294 L295 L296 L297 L298 L299 | L490 L687 L689 L690 L699 L700 L701 L702 L703 L704 | L9 L1075 L1274 L1275 L1284 L1285 L1286 L1287 L1288 L1289 | L880 L1077 L1079 L1080 L1089 L1090 L1091 L1092 L1093 L1094 | L685 L882 L884 L885 L894 L895 L896 L897 L898 L899 | L6 L102 L104 L105 L114 L115 L116 L117 L118 L119 | L100 L297 L299 L300 L309 L310 L311 L312 L313 L314 | L295 L492 L494 L495 L504 L505 L506 L507 L508 L509 | L505 L702 L704 L705 L714 L715 L716 L717 L718 L719 | L9 L1285 L1484 L1485 L1494 L1495 L1496 L1497 L1498 L1499 | L1090 L1287 L1289 L1290 L1299 L1300 L1301 L1302 L1303 L1304 | L895 L1092 L1094 L1095 L1104 L1105 L1106 L1107 L1108 L1109 | L700 L897 L899 L900 L909 L910 L911 L912 L913 L914 | L6 L117 L119 L120 L129 L130 L131 L132 L133 L134 | L115 L312 L314 L315 L324 L325 L326 L327 L328 L329 | L310 L507 L509 L510 L519 L520 L521 L522 L523 L524 | L715 L912 L914 L915 L924 L925 L926 L927 L928 L929 | L9 L1495 L1694 L1695 L1704 L1705 L1706 L1707 L1708 L1709 | L1300 L1497 L1499 L1500 L1509 L1510 L1511 L1512 L1513 L1514 | L1105 L1302 L1304 L1305 L1314 L1315 L1316 L1317 L1318 L1319 | L910 L1107 L1109 L1110 L1119 L1120 L1121 L1122 L1123 L1124 | L6 L132 L134 L135 L144 L145 L146 L147 L148 L149 | L130 L327 L329 L330 L339 L340 L341 L342 L343 L344 | L325 L522 L524 L525 L534 L535 L536 L537 L538 L539 | L520 L717 L719 L720 L729 L730 L731 L732 L733 L734 | L730 L927 L929 L930 L939 L940 L941 L942 L943 L944 | L9 L1705 L1904 L1905 L1914 L1915 L1916 L1917 L1918 L1919 | L1510 L1707 L1709 L1710 L1719 L1720 L1721 L1722 L1723 L1724 | L1315 L1512 L1514 L1515 L1524 L1525 L1526 L1527 L1528 L1529 | L1120 L1317 L1319 L1320 L1329 L1330 L1331 L1332 L1333 L1334 | L925 L1122 L1124 L1125 L1134 L1135 L1136 L1137 L1138 L1139 | L6 L147 L149 L150 L159 L160 L161 L162 L163 L164 | L145 L342 L344 L345 L354 L355 L356 L357 L358 L359 | L340 L537 L539 L540 L549 L550 L551 L552 L553 L554 | L535 L732 L734 L735 L744 L745 L746 L747 L748 L749 | L940 L1137 L1139 L1140 L1149 L1150 L1151 L1152 L1153 L1154 | L9 L1915 L2114 L2115 L2124 L2125 L2126 L2127 L2128 L2129 | L1720 L1917 L1919 L1920 L1929 L1930 L1931 L1932 L1933 L1934 | L1525 L1722 L1724 L1725 L1734 L1735 L1736 L1737 L1738 L1739 | L1330 L1527 L1529 L1530 L1539 L1540 L1541 L1542 L1543 L1544 | L1135 L1332 L1334 L1335 L1344 L1345 L1346 L1347 L1348 L1349 | L6 L162 L164 L165 L174 L175 L176 L177 L178 L179 | L160 L357 L359 L360 L369 L370 L371 L372 L373 L374 | L355 L552 L554 L555 L564 L565 L566 L567 L568 L569 | L550 L747 L749 L750 L759 L760 L761 L762 L763 L764 | L745 L942 L944 L945 L954 L955 L956 L957 L958 L959 | L955 L1152 L1154 L1155 L1164 L1165 L1166 L1167 L1168 L1169 | L9 L2125 L2324 L2325 L2334 L2335 L2336 L2337 L2338 L2339 | L1930 L2127 L2129 L2130 L2139 L2140 L2141 L2142 L2143 L2144 | L1735 L1932 L1934 L1935 L1944 L1945 L1946 L1947 L1948 L1949 | L1540 L1737 L1739 L1740 L1749 L1750 L1751 L1752 L1753 L1754 | L1345 L1542 L1544 L1545 L1554 L1555 L1556 L1557 L1558 L1559 | L1150 L1347 L1349 L1350 L1359 L1360 L1361 L1362 L1363 L1364 | L6 L177 L179 L180 L189 L190 L191 L192 L193 L194 | L175 L372 L374 L375 L384 L385 L386 L387 L388 L389 | L370 L567 L569 L570 L579 L580 L581 L582 L583 L584 | L565 L762 L764 L765 L774 L775 L776 L777 L778 L779 | L760 L957 L959 L960 L969 L970 L971 L972 L973 L974 | L1165 L1362 L1364 L1365 L1374 L1375 L1376 L1377 L1378 L1379 | L9 L2335 L2534 L2535 L2544 L2545 L2546 L2547 L2548 L2549 | L2140 L2337 L2339 L2340 L2349 L2350 L2351 L2352 L2353 L2354 | L1945 L2142 L2144 L2145 L2154 L2155 L2156 L2157 L2158 L2159 | L1750 L1947 L1949 L1950 L1959 L1960 L1961 L1962 L1963 L1964 | L1555 L1752 L1754 L1755 L1764 L1765 L1766 L1767 L1768 L1769 | L1360 L1557 L1559 L1560 L1569 L1570 L1571 L1572 L1573 L1574 | L6 L192 L194 L195 L204 L205 L206 L207 L208 L209 | L190 L387 L389 L390 L399 L400 L401 L402 L403 L404 | L385 L582 L584 L585 L594 L595 L596 L597 L598 L599 | L580 L777 L779 L780 L789 L790 L791 L792 L793 L794 | L775 L972 L974 L975 L984 L985 L986 L987 L988 L989 | L970 L1167 L1169 L1170 L1179 L1180 L1181 L1182 L1183 L1184 | L1180 L1377 L1379 L1380 L1389 L1390 L1391 L1392 L1393 L1394 | L8 L9 L2545 L2744 L2745 L2754 L2755 L2756 L2757 L2758 L2759 | L2350 L2547 L2549 L2550 L2559 L2560 L2561 L2562 L2563 L2564 | L2155 L2352 L2354 L2355 L2364 L2365 L2366 L2367 L2368 L2369 | L1960 L2157 L2159 L2160 L2169 L2170 L2171 L2172 L2173 L2174 | L1765 L1962 L1964 L1965 L1974 L1975 L1976 L1977 L1978 L1979 | L1570 L1767 L1769 L1770 L1779 L1780 L1781 L1782 L1783 L1784 | L1375 L1572 L1574 L1575 L1584 L1585 L1586 L1587 L1588 L1589 | L6 L7 L207 L209 L210 L219 L220 L221 L222 L223 | L205 L402 L404 L405 L414 L415 L416 L417 L418 L419 | L400 L597 L599 L600 L609 L610 L611 L612 L613 L614 | L595 L792 L794 L795 L804 L805 L806 L807 L808 L809 | L790 L987 L989 L990 L999 L1000 L1001 L1002 L1003 L1004 | L985 L1182 L1184 L1185 L1194 L1195 L1196 L1197 L1198 L1199 | L1390 L1587 L1589 L1590 L1599 L1600 L1601 L1602 L1603 L1604 | L8 L2560 L2757 L2759 L2760 L2769 L2770 L2771 L2772 L2773 L2774 | L2365 L2562 L2564 L2565 L2574 L2575 L2576 L2577 L2578 L2579 | L2170 L2367 L2369 L2370 L2379 L2380 L2381 L2382 L2383 L2384 | L1975 L2172 L2174 L2175 L2184 L2185 L2186 L2187 L2188 L2189 | L1780 L1977 L1979 L1980 L1989 L1990 L1991 L1992 L1993 L1994 | L1585 L1782 L1784 L1785 L1794 L1795 L1796 L1797 L1798 L1799 | L7 L220 L417 L419 L420 L429 L430 L431 L432 L433 | L415 L612 L614 L615 L624 L625 L626 L627 L628 L629 | L610 L807 L809 L810 L819 L820 L821 L822 L823 L824 | L805 L1002 L1004 L1005 L1014 L1015 L1016 L1017 L1018 L1019 | L1000 L1197 L1199 L1200 L1209 L1210 L1211 L1212 L1213 L1214 | L1195 L1392 L1394 L1395 L1404 L1405 L1406 L1407 L1408 L1409 | L1405 L1602 L1604 L1605 L1614 L1615 L1616 L1617 L1618 L1619 | L8 L2575 L2772 L2774 L2775 L2784 L2785 L2786 L2787 L2788 L2789 | L2380 L2577 L2579 L2580 L2589 L2590 L2591 L2592 L2593 L2594 | L2185 L2382 L2384 L2385 L2394 L2395 L2396 L2397 L2398 L2399 | L1990 L2187 L2189 L2190 L2199 L2200 L2201 L2202 L2203 L2204 | L1795 L1992 L1994 L1995 L2004 L2005 L2006 L2007 L2008 L2009 | L1600 L1797 L1799 L1800 L1809 L1810 L1811 L1812 L1813 L1814 | L7 L430 L627 L629 L630 L639 L640 L641 L642 L643 | L625 L822 L824 L825 L834 L835 L836 L837 L838 L839 | L820 L1017 L1019 L1020 L1029 L1030 L1031 L1032 L1033 L1034 | L1015 L1212 L1214 L1215 L1224 L1225 L1226 L1227 L1228 L1229 | L1210 L1407 L1409 L1410 L1419 L1420 L1421 L1422 L1423 L1424 | L1615 L1812 L1814 L1815 L1824 L1825 L1826 L1827 L1828 L1829 | L8 L2590 L2787 L2789 L2790 L2799 L2800 L2801 L2802 L2803 L2804 | L2395 L2592 L2594 L2595 L2604 L2605 L2606 L2607 L2608 L2609 | L2200 L2397 L2399 L2400 L2409 L2410 L2411 L2412 L2413 L2414 | L2005 L2202 L2204 L2205 L2214 L2215 L2216 L2217 L2218 L2219 | L1810 L2007 L2009 L2010 L2019 L2020 L2021 L2022 L2023 L2024 | L7 L640 L837 L839 L840 L849 L850 L851 L852 L853 | L835 L1032 L1034 L1035 L1044 L1045 L1046 L1047 L1048 L1049 | L1030 L1227 L1229 L1230 L1239 L1240 L1241 L1242 L1243 L1244 | L1225 L1422 L1424 L1425 L1434 L1435 L1436 L1437 L1438 L1439 | L1420 L1617 L1619 L1620 L1629 L1630 L1631 L1632 L1633 L1634 | L1630 L1827 L1829 L1830 L1839 L1840 L1841 L1842 L1843 L1844 | L8 L2605 L2802 L2804 L2805 L2814 L2815 L2816 L2817 L2818 L2819 | L2410 L2607 L2609 L2610 L2619 L2620 L2621 L2622 L2623 L2624 | L2215 L2412 L2414 L2415 L2424 L2425 L2426 L2427 L2428 L2429 | L2020 L2217 L2219 L2220 L2229 L2230 L2231 L2232 L2233 L2234 | L1825 L2022 L2024 L2025 L2034 L2035 L2036 L2037 L2038 L2039 | L7 L850 L1047 L1049 L1050 L1059 L1060 L1061 L1062 L1063 | L1045 L1242 L1244 L1245 L1254 L1255 L1256 L1257 L1258 L1259 | L1240 L1437 L1439 L1440 L1449 L1450 L1451 L1452 L1453 L1454 | L1435 L1632 L1634 L1635 L1644 L1645 L1646 L1647 L1648 L1649 | L1840 L2037 L2039 L2040 L2049 L2050 L2051 L2052 L2053 L2054 | L8 L2620 L2817 L2819 L2820 L2829 L2830 L2831 L2832 L2833 L2834 | L2425 L2622 L2624 L2625 L2634 L2635 L2636 L2637 L2638 L2639 | L2230 L2427 L2429 L2430 L2439 L2440 L2441 L2442 L2443 L2444 | L2035 L2232 L2234 L2235 L2244 L2245 L2246 L2247 L2248 L2249 | L7 L1060 L1257 L1259 L1260 L1269 L1270 L1271 L1272 L1273 | L1255 L1452 L1454 L1455 L1464 L1465 L1466 L1467 L1468 L1469 | L1450 L1647 L1649 L1650 L1659 L1660 L1661 L1662 L1663 L1664 | L1645 L1842 L1844 L1845 L1854 L1855 L1856 L1857 L1858 L1859 | L1855 L2052 L2054 L2055 L2064 L2065 L2066 L2067 L2068 L2069 | L8 L2635 L2832 L2834 L2835 L2844 L2845 L2846 L2847 L2848 L2849 | L2440 L2637 L2639 L2640 L2649 L2650 L2651 L2652 L2653 L2654 | L2245 L2442 L2444 L2445 L2454 L2455 L2456 L2457 L2458 L2459 | L2050 L2247 L2249 L2250 L2259 L2260 L2261 L2262 L2263 L2264 | L7 L1270 L1467 L1469 L1470 L1479 L1480 L1481 L1482 L1483 | L1465 L1662 L1664 L1665 L1674 L1675 L1676 L1677 L1678 L1679 | L1660 L1857 L1859 L1860 L1869 L1870 L1871 L1872 L1873 L1874 | L2065 L2262 L2264 L2265 L2274 L2275 L2276 L2277 L2278 L2279 | L8 L2650 L2847 L2849 L2850 L2859 L2860 L2861 L2862 L2863 L2864 | L2455 L2652 L2654 L2655 L2664 L2665 L2666 L2667 L2668 L2669 | L2260 L2457 L2459 L2460 L2469 L2470 L2471 L2472 L2473 L2474 | L7 L1480 L1677 L1679 L1680 L1689 L1690 L1691 L1692 L1693 | L1675 L1872 L1874 L1875 L1884 L1885 L1886 L1887 L1888 L1889 | L1870 L2067 L2069 L2070 L2079 L2080 L2081 L2082 L2083 L2084 | L2080 L2277 L2279 L2280 L2289 L2290 L2291 L2292 L2293 L2294 | L8 L2665 L2862 L2864 L2865 L2874 L2875 L2876 L2877 L2878 L2879 | L2470 L2667 L2669 L2670 L2679 L2680 L2681 L2682 L2683 L2684 | L2275 L2472 L2474 L2475 L2484 L2485 L2486 L2487 L2488 L2489 | L7 L1690 L1887 L1889 L1890 L1899 L1900 L1901 L1902 L1903 | L1885 L2082 L2084 L2085 L2094 L2095 L2096 L2097 L2098 L2099 | L2290 L2487 L2489 L2490 L2499 L2500 L2501 L2502 L2503 L2504 | L8 L2680 L2877 L2879 L2880 L2889 L2890 L2891 L2892 L2893 L2894 | L2485 L2682 L2684 L2685 L2694 L2695 L2696 L2697 L2698 L2699 | L7 L1900 L2097 L2099 L2100 L2109 L2110 L2111 L2112 L2113 | L2095 L2292 L2294 L2295 L2304 L2305 L2306 L2307 L2308 L2309 | L2305 L2502 L2504 L2505 L2514 L2515 L2516 L2517 L2518 L2519 | L8 L2695 L2892 L2894 L2895 L2904 L2905 L2906 L2907 L2908 L2909 | L2500 L2697 L2699 L2700 L2709 L2710 L2711 L2712 L2713 L2714 | L7 L2110 L2307 L2309 L2310 L2319 L2320 L2321 L2322 L2323 | L2515 L2712 L2714 L2715 L2724 L2725 L2726 L2727 L2728 L2729 | L8 L2710 L2907 L2909 L2910 L2919 L2920 L2921 L2922 L2923 L2924 | L7 L2320 L2517 L2519 L2520 L2529 L2530 L2531 L2532 L2533 | L7 L2530 L2727 L2729 L2730 L2739 L2740 L2741 L2742 L2743 | L8 L2725 L2922 L2924 L2925 L2934 L2935 L2936 L2937 L2938 L2939 | L7 L8 L2740 L2937 L2939 L2940 L2949 L2950 L2951 L2952 L2953